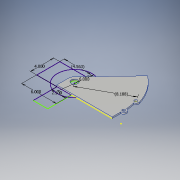
# Autodesk Inventor part: Hood panel RIGHT
Saved by Autodesk Inventor 2018 (Build 220112000, 112)
## iProperties
Created: 2020-01-18
Part Number: Hood panel RIGHT
Material: Aluminum 6061
Document SubType Name: Modeling
Designer: Victor
Density: 2.7 g/cm^3
Appearance: Aluminum - Flat
Author: Victor
Autodesk Inventor part; units mm, degrees
ref_plane "YZ Plane" through (0, 0, 0) normal (1, 0, 0) x (0, 1, 0)
ref_plane "XZ Plane" through (0, 0, 0) normal (0, 1, 0) x (-1, 0, 0)
ref_plane "XY Plane" through (0, 0, 0) normal (0, 0, 1) x (1, 0, 0)
sketch "Sketch1" plane through (0, 0, 0) normal (0, 1, 0) x (-1, 0, 0)
  circle A0 centre (254, -50.8) radius 14.2875
  arc A1 (38.4735, -38.1055) -> (38.4735, -63.4945) centre (38.1, -50.8) ccw
  line L0 (280.9875, -50.8) -> (280.9875, 0)
  line L1 (280.9875, 0) -> (280.9875, -50.8)
  line L2 (280.9875, 0) -> (38.1, 0)
  line L3 (38.1, -38.1) -> (38.1, 0)
  arc A2 (38.4735, -63.4945) -> (43.8871, -100.4525) centre (254, -50.8) ccw
  arc A3 (51.1687, -124.7749) -> (66.9545, -158.6276) centre (254, -50.8) ccw
  arc A4 (80.906, -179.8398) -> (105.7377, -207.743) centre (254, -50.8) ccw
  arc A5 (273.4803, -69.4773) -> (280.9875, -50.8) centre (254, -50.8) ccw
  line L4 (125.2338, -224.0976) -> (273.4803, -69.4773)
  line L5 (280.9875, 0) -> (38.1, 0)
  line L6 (38.1, 0) -> (38.1, -38.1)
  line L7 (280.9875, 0) -> (280.9875, -50.8)
  circle A6 centre (47.1701, -112.7208) radius 6.35
  circle A7 centre (38.1, -50.8) radius 6.35
  arc A8 (43.8871, -100.4525) -> (51.1687, -124.7749) centre (47.1701, -112.7208) ccw
  arc A9 (38.4735, -38.1055) -> (38.4735, -63.4945) centre (38.1, -50.8) ccw
  arc A10 (43.8871, -100.4525) -> (51.1687, -124.7749) centre (47.1701, -112.7208) ccw
  line L8 (38.1, 0) -> (50.8, 0)
  line L9 (38.4739, -38.1) -> (38.1, -38.1)
  line L10 (38.1, -38.1) -> (38.1, 0)
  circle A11 centre (254, -50.8) radius 14.2875
  circle A12 centre (47.1701, -112.7208) radius 6.35
  circle A13 centre (38.1, -50.8) radius 6.35
  arc A14 (51.1687, -124.7749) -> (125.2338, -224.0976) centre (254, -50.8) ccw
  arc A15 (38.1934, -57.1493) -> (43.8871, -100.4525) centre (254, -50.8) ccw
  arc A16 (35.0036, -116.3632) -> (116.3789, -233.3332) centre (254, -50.8) ccw
  line L11 (125.2338, -224.0976) -> (116.3789, -233.3332)
  point P0 (0, 0)
  point P1 (44.1616, 0)
  point P2 (38.1934, -44.4507)
  dimension "d4" = 28.575
  dimension "d32" = 25.4
  dimension "d36" = 50.8
  dimension "d74" = 53.975
  dimension "d79" = 12.7
  dimension "d83" = 26.9875
  constraints: 28 point on circle, 24 end point, 17 centre point, 10 coincident, 3 collinear, 2 horizontal, 2 tangent, 1 parallel, 1 perpendicular, 1 point on line, 1 vertical
  measures "d4" diameter of A0
  measures "d32" diameter of A1
  measures "d36" distance of L0.start L0.end
  measures "d74" diameter of A5
  measures "d79" diameter of A7
  measures "d83" distance from line of L0 A0.centre
ref_plane "Work Plane1" through (0, 6.35, 0) normal (0, 1, 0) x (1, 0, 0)
extrude "Extrusion7" add sketch "Sketch1" along normal blind 6.35
sketch "Sketch3" plane through (0, 0, 0) normal (0, -1, 0) x (1, 0, 0)
  circle A0 centre (-254, -50.8) radius 14.2875 projected
  circle A1 centre (-254, -50.8) radius 14.2875
  arc A2 (-116.3789, -233.3332) -> (-35.0036, -116.3632) centre (-254, -50.8) ccw projected
  circle A3 centre (-47.1701, -112.7208) radius 6.35 projected
  arc A4 (-130.7722, -218.3211) -> (-55.5923, -113.1119) centre (-254, -50.8) ccw
  circle A5 centre (-254, -50.8) radius 24.789
  arc A6 (-126.3412, -222.9426) -> (-47.018, -106.3726) centre (-254, -50.8) ccw
  arc A7 (-54.9513, -130.2322) -> (-60.849, -127.8786) centre (-57.9002, -129.0554) ccw
  line L0 (-62.5231, -105.8831) -> (-35.6006, -133.9631)
  line L1 (-116.3789, -233.3332) -> (-273.4803, -69.4773) projected
  arc A8 (-120.5628, -210.3083) -> (-116.4883, -215.1788) centre (-118.5256, -212.7436) ccw
  arc A9 (-56.7456, -126.0977) -> (-50.5804, -107.3643) centre (-254, -50.8) ccw
  arc A10 (-128.5564, -220.6321) -> (-120.976, -214.7624) centre (-254, -50.8) ccw
  point P0 (0, 0)
  dimension "d90" = 415.925
  dimension "d94" = 428.625
  dimension "d97" = 6.35
  dimension "d98" = 6.35
  dimension "d101" = 12.7
  dimension "d102" = 6.35
  dimension "d103" = 12.7
  constraints: 20 point on circle, 8 centre point, 4 point on line, 3 tangent, 2 coincident, 2 end point, 1 concentric, 1 parallel
  measures "d90" diameter of A4
  measures "d94" diameter of A6
  measures "d97" radial gap between concentric circles of A4 A6
  measures "d98" diameter of A7
  measures "d101" distance from line of L0 A7.centre
  measures "d102" diameter of A8
  measures "d103" distance from line of L1 A8.centre
extrude "Extrusion8" cut sketch "Sketch3" against normal blind 3.175 contours A8 A4 A7 A6
sketch "Sketch5" plane through (0, 3.175, 0) normal (0, -1, 0) x (1, 0, 0)
  arc A0 (-120.5628, -210.3083) -> (-116.4883, -215.1788) centre (-118.5256, -212.7436) ccw projected
  circle A1 centre (-118.5256, -212.7436) radius 3.175
  point P0 (0, 0)
  constraints: 1 coincident, 3 other
extrude "Extrusion9" add sketch "Sketch5" along normal blind 19.05
sketch "Sketch6" plane through (-118.5256, -15.875, -212.7436) normal (0, -1, 0) x (1, 0, 0)
  arc A0 (-2.0372, 2.4352) -> (2.0372, -2.4352) centre (0, 0) ccw projected
  circle A1 centre (0, 0) radius 6.35
  point P0 (118.5256, 212.7436)
  dimension "d108" = 12.7
  constraints: 1 centre point, 1 coincident
  measures "d108" diameter of A1
extrude "Extrusion10" add sketch "Sketch6" against normal blind 6.35
sketch "Sketch7" plane through (0, 0, 0) normal (0, -1, 0) x (1, 0, 0)
  line L0 (-280.9875, 0) -> (-38.1, 0) projected
  line L1 (-217.4875, 0) -> (-369.8875, 0)
  line L2 (-369.8875, 0) -> (-369.8875, -101.6)
  line L3 (-369.8875, -101.6) -> (-217.4875, -101.6)
  line L4 (-217.4875, -101.6) -> (-217.4875, 0)
  line L5 (-280.9875, -50.8) -> (-280.9875, 0) projected
  line L6 (-116.3789, -233.3332) -> (-273.4803, -69.4773) projected
  line L7 (-242.6818, -101.6) -> (-276.2977, -52.4082)
  line L8 (-276.2977, -52.4082) -> (-253.5984, 0)
  circle A0 centre (-254, -50.8) radius 14.2875 projected
  circle A1 centre (-254, -50.8) radius 14.2875
  line L9 (-280.9875, 0) -> (-217.4875, 0)
  line L10 (-217.4875, 0) -> (-217.4875, 104.2647)
  line L11 (-217.4875, 104.2647) -> (-280.9875, 104.2647)
  line L12 (-280.9875, 104.2647) -> (-280.9875, 0)
  circle A2 centre (-254, -50.8) radius 76.2
  circle A3 centre (-47.1701, -112.7208) radius 6.35 projected
  line L13 (-254, -50.8) -> (-71.9918, -151.4053)
  arc A4 (-120.5628, -210.3083) -> (-60.849, -127.8786) centre (-254, -50.8) ccw projected
  point P0 (0, 0)
  dimension "d111" = 63.5
  dimension "d112" = 101.6
  dimension "d113" = 152.4
  dimension "d114" = 115.8875
  dimension "d115" = 152.4
  dimension "d118" = 207.9625
  constraints: 22 end point, 4 parallel, 4 point on line, 2 centre point, 2 coincident, 2 horizontal, 2 perpendicular, 1 point on circle
  measures "d111" distance between parallel lines of L5 L4
  measures "d112" distance between parallel lines of L0 L3
  measures "d113" distance of L1.start L1.end
  measures "d114" distance from line of L2 A1.centre
  measures "d115" diameter of A2
  measures "d118" distance of L13.start L13.end
body "Solid4"
